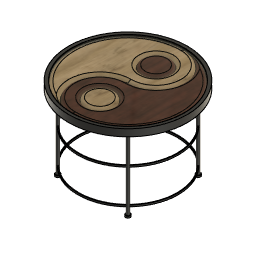
Yin+and+Yang+Table (Autodesk Fusion 360 design; units mm, degrees)
Autodesk Fusion 360 part; units mm, degrees
sketch "Sketch1" plane through (0, 0, 0) normal (0, 0, 1) x (1, 0, 0)
  circle A0 centre (0, 0) radius 457.2
  circle A1 centre (0, -228.6) radius 114.3
  circle A2 centre (0, 228.6) radius 114.3
  arc A3 (0, 0) -> (0, 457.2) centre (0, 228.6) ccw
  arc A4 (0, 0) -> (0, -457.2) centre (0, -228.6) ccw
  dimension "d5" = 457.2
  dimension "d6" = 457.2
  dimension "d7" = 228.6
  dimension "d8" = 228.6
  dimension "d9" = 228.6
  dimension "d10" = 228.6
  dimension "d11" = 914.4
  dimension "d12" = 228.6
  dimension "d13" = 228.6
  constraint coincident A0.centre A3.start
  constraint concentric A1 A4
  constraint concentric A2 A3
  constraint coincident A0 A3.end
  constraint coincident A0.centre A4
  constraint coincident A0 A4.end
  constraint coincident A3 A0.centre
  measures "d5" diameter of A3
  measures "d6" diameter of A4
  measures "d7" diameter of A1
  measures "d8" diameter of A2
  measures "d9" distance of A0.centre A2.centre
  measures "d10" distance of A0.centre A1.centre
  measures "d11" diameter of A0
  measures "d12" radius of A4
  measures "d13" radius of A3
extrude "Extrude1" add sketch "Sketch1" along normal blind 50.8 contours A0 A3 A4 | A1 picked at (-228.0212, 95.0056) makes body 1 at (-228.0212, 95.0056, 0) makes body 2 at (-59.3187, -250.0625, 0) in component "Component"
extrude "Extrude1'" add sketch "Sketch1" along normal blind 50.8 separate body contours A0 A3 A4 | A2 picked at (232.3828, -82.2636) makes body 3 at (228.0212, -95.0056, 0) makes body 4 at (35.0802, 259.2365, 0) in component "Component'"
fillet "Fillet1" radius 25.4 2 faces at (228.0212, -95.0056, 50.8) (35.0802, 259.2365, 50.8) on bodies 3 4 in component "Component'"
fillet "Fillet1'" radius 25.4 2 faces at (-228.0212, 95.0056, 50.8) (-59.3187, -250.0625, 50.8) on bodies 1 2 in component "Component"
sketch "Sketch2" plane through (0, 0, 0) normal (0, 0, 1) x (1, 0, 0)
  circle A0 centre (0, 0) radius 457.2
  circle A1 centre (0, 0) radius 482.6
  circle A2 centre (0, 0) radius 469.9
  dimension "d29" = 914.4
  dimension "d30" = 25.4
  dimension "d31" = 12.7
  constraint coincident A0.centre A1.centre
  measures "d29" diameter of A0
extrude "Extrude3" add sketch "Sketch2" along normal blind 57.15 separate body contours A1 | A2 makes body 5
extrude "Extrude4" add sketch "Sketch2" against normal blind 5.08 separate body contours A0 | A2 makes body 6
sketch "Sketch3" plane through (0, 0, 0) normal (0, 0, 1) x (1, 0, 0)
  circle A0 centre (0, 0) radius 457.2
  circle A1 centre (0, 0) radius 457.2
  line L0 (0, -457.2) -> (395.9468, -228.6)
  line L1 (395.9468, -228.6) -> (395.9468, 228.6)
  line L2 (395.9468, 228.6) -> (0, 457.2)
  line L3 (0, 457.2) -> (-395.9468, 228.6)
  line L4 (-395.9468, 228.6) -> (-395.9468, -228.6)
  line L5 (-395.9468, -228.6) -> (0, -457.2)
  line L6 (-370.5468, -213.9353) -> (0, -427.8706)
  line L7 (0, -427.8706) -> (370.5468, -213.9353)
  line L8 (370.5468, -213.9353) -> (370.5468, 213.9353)
  line L9 (370.5468, 213.9353) -> (0, 427.8706)
  line L10 (0, 427.8706) -> (-370.5468, 213.9353)
  line L11 (-370.5468, 213.9353) -> (-370.5468, -213.9353)
  line L12 (-345.1468, 199.2706) -> (-345.1468, -199.2706)
  line L13 (-345.1468, -199.2706) -> (0, -398.5412)
  line L14 (0, -398.5412) -> (345.1468, -199.2706)
  line L15 (345.1468, -199.2706) -> (345.1468, 199.2706)
  line L16 (345.1468, 199.2706) -> (0, 398.5412)
  line L17 (0, 398.5412) -> (-345.1468, 199.2706)
  line L18 (0, -50.8) -> (43.9941, -25.4)
  line L19 (43.9941, -25.4) -> (43.9941, 25.4)
  line L20 (43.9941, 25.4) -> (0, 50.8)
  line L21 (0, 50.8) -> (-43.9941, 25.4)
  line L22 (-43.9941, 25.4) -> (-43.9941, -25.4)
  line L23 (-43.9941, -25.4) -> (0, -50.8)
  dimension "d36" = 914.4
  dimension "d37" = 914.4
  dimension "d38" = -25.4
  dimension "d39" = -50.8
  dimension "d46" = 50.8
  constraint coincident A0.centre A1.centre
  constraint coincident A0 L0.start
  measures "d36" diameter of A0
  measures "d37" diameter of A1
  measures "d46" distance of L18.start A0.centre
extrude "Extrude5" add sketch "Sketch3" against normal blind 25.4 separate body contours L6 L7 L8 L9 L10 L11 makes body 7
sketch "Sketch4" plane through (0, 0, 0) normal (0, 0, 1) x (1, 0, 0)
  circle A0 centre (0, 0) radius 457.2
  line L0 (323.2892, 323.2892) -> (-323.2892, 323.2892)
  line L1 (-323.2892, 323.2892) -> (-323.2892, -323.2892)
  line L2 (-323.2892, -323.2892) -> (323.2892, -323.2892)
  line L3 (323.2892, -323.2892) -> (323.2892, 323.2892)
  line L4 (323.2892, 323.2892) -> (-323.2892, -323.2892) construction
  line L5 (-323.2892, 323.2892) -> (323.2892, -323.2892) construction
  dimension "d42" = 914.4
  dimension "d43" = 90
  constraint coincident A0.centre origin
  constraint horizontal L0
  constraint perpendicular L0 L1
  constraint parallel L0 L2
  constraint parallel L1 L3
  constraint coincident L4 A0.centre
  constraint coincident L5 A0.centre
  constraint coincident A0 L0.start
  measures "d42" diameter of A0
  measures "d43" angle of L4 L5
sketch "Sketch5" plane through (0, 0, 0) normal (0, 0, 1) x (1, 0, 0)
  circle A0 centre (0, 0) radius 457.2
  line L0 (0, 0) -> (-482.6, 0) construction
  dimension "d44" = 914.4
  constraint coincident A0.centre L0.start
  constraint horizontal L0
  measures "d44" diameter of A0
extrude "Extrude6" add sketch "Sketch3" against normal blind 609.6 separate body contours L18 L19 L20 L21 L22 L23 makes body 8
sketch "Sketch6" plane through (0, 0, 0) normal (0, 0, 1) x (1, 0, 0)
  line L0 (285.75, -285.75, -5.08) -> (-285.75, -285.75, -5.08)
  line L1 (-285.75, -285.75, -5.08) -> (-285.75, 285.75, -5.08)
  line L2 (-285.75, 285.75, -5.08) -> (285.75, 285.75, -5.08)
  line L3 (285.75, 285.75, -5.08) -> (285.75, -285.75, -5.08)
  line L4 (285.75, -285.75, -5.08) -> (-285.75, 285.75, -5.08) construction
  line L5 (-285.75, -285.75, -5.08) -> (285.75, 285.75, -5.08) construction
  line L6 (-285.75, 285.75, -5.08) -> (-260.35, 285.75, -5.08)
  line L7 (-260.35, 285.75, -5.08) -> (-260.35, 260.35, -5.08)
  line L8 (-260.35, 260.35, -5.08) -> (-285.75, 260.35, -5.08)
  line L9 (-285.75, 260.35, -5.08) -> (-285.75, 285.75, -5.08)
  line L10 (285.75, 285.75, -5.08) -> (260.35, 285.75, -5.08)
  line L11 (260.35, 285.75, -5.08) -> (260.35, 260.35, -5.08)
  line L12 (260.35, 260.35, -5.08) -> (285.75, 260.35, -5.08)
  line L13 (285.75, 260.35, -5.08) -> (285.75, 285.75, -5.08)
  line L14 (-285.75, -285.75, -5.08) -> (-212.2467, -285.75, -5.08)
  line L15 (-212.2467, -285.75, -5.08) -> (-212.2467, -212.2467, -5.08)
  line L16 (-212.2467, -212.2467, -5.08) -> (-285.75, -212.2467, -5.08)
  line L17 (-285.75, -212.2467, -5.08) -> (-285.75, -285.75, -5.08)
  line L18 (285.75, -285.75, -5.08) -> (210.9673, -285.75, -5.08)
  line L19 (210.9673, -285.75, -5.08) -> (210.9673, -210.9673, -5.08)
  line L20 (210.9673, -210.9673, -5.08) -> (285.75, -210.9673, -5.08)
  line L21 (285.75, -210.9673, -5.08) -> (285.75, -285.75, -5.08)
  circle A0 through (-273.05, -285.75, -5.08) (-292.1, -274.7515, -5.08) (-292.1, -296.7485, -5.08)
  circle A1 through (298.45, -285.75, -5.08) (279.4, -274.7515, -5.08) (279.4, -296.7485, -5.08)
  circle A2 through (-273.05, 285.75, -5.08) (-292.1, 296.7485, -5.08) (-292.1, 274.7515, -5.08)
  circle A3 through (298.45, 285.75, -5.08) (279.4, 296.7485, -5.08) (279.4, 274.7515, -5.08)
  circle A4 through (469.9, 0, -5.08) (-234.95, 406.9453, -5.08) (-234.95, -406.9453, -5.08)
  circle A5 centre (0, 0) radius 404.1115
  circle A6 centre (0, 0) radius 407.2865
  circle A7 centre (0, 0) radius 400.9365
  dimension "d49" = 571.5
  dimension "d50" = 571.5
  dimension "d51" = 25.4
  dimension "d52" = 25.4
  dimension "d53" = 25.4
  dimension "d54" = 25.4
  dimension "d55" = 25.4
  dimension "d59" = 25.4
  dimension "d60" = 25.4
  dimension "d62" = 25.4
  dimension "d68" = 3.175
  dimension "d69" = -3.175
  constraint coincident A5.centre A6.centre
extrude "Extrude1''" add sketch "Sketch6" against normal blind 609.6 separate body contours L0 L3 L18 L21 A1 | L0 L3 L18 L21 A1 | L0 L1 L14 L17 A0 | L0 L1 L14 L17 A0 | L2 L3 L10 L13 A3 | L2 L3 L10 L13 A3 | L1 L2 L6 L9 A2 | L1 L2 L6 L9 A2 in plane through (0, 0, -5.08) normal (0, 0, 1) makes body 9 at (298.0573, -288.8838, -208.28) makes body 10 at (-273.3018, -283.2335, -411.48) makes body 11 at (298.1982, 288.2665, -411.48) makes body 12 at (-273.3018, 288.2665, -411.48) in component "Component''"
copy_body "Body->Comp1" bodies 5 removing the originals makes body 13 in component "Component'''"
copy_body "CutPasteBodies1" bodies 6 removing the originals makes body 14 in component "Component'''"
sketch "Sketch7" plane through (0, 0, 57.15) normal (0, 0, 1) x (-1, 0, 0)
  circle A0 centre (0, 0) radius 457.2
  circle A1 centre (0, 0) radius 482.6
  circle A2 centre (0, 0) radius 457.2
extrude "Extrude7" add sketch "Sketch7" against normal blind 7.9375 from surface at -1.524 separate body contours A0 A2 makes body 15
sketch "Sketch8" plane through (0, 0, -614.68) normal (0, 0, -1) x (1, 0, 0)
  circle A0 centre (-285.75, -285.75) radius 12.7
  circle A1 centre (-285.75, -285.75) radius 19.05
  dimension "d65" = 38.1
  constraint concentric A0 A1
  measures "d65" diameter of A1
extrude "Extrude8" add sketch "Sketch8" against normal blind 12.7 separate body makes body 16
copy_body "CopyPasteBodies1" bodies 16 makes body 17
move_body "Move1" bodies 17 to x (1, 0, 0) y (0, 1, 0) z (0, 0, 1) at (0, -571.5, 0)
copy_body "CopyPasteBodies2" bodies 16 makes body 18
move_body "Move2" bodies 18 to x (1, 0, 0) y (0, 1, 0) z (0, 0, 1) at (571.5, -571.5, 0)
copy_body "CopyPasteBodies3" bodies 16 makes body 19
move_body "Move3" bodies 19 to x (1, 0, 0) y (0, 1, 0) z (0, 0, 1) at (571.5, 0, 0)
sketch "Sketch9" plane through (0, 0, 0) normal (0, 0, 1) x (1, 0, 0)
  circle A0 centre (0, 0) radius 407.2865
  circle A1 centre (0, 0) radius 404.1115
  circle A2 centre (0, 0) radius 400.9365
  dimension "d70" = 3.175
  dimension "d71" = -3.175
extrude "Extrude9" add sketch "Sketch9" against normal blind 12.7 from surface at -304.8 separate body contours A0 | A1 makes body 20
copy_body "CopyPasteBodies4" bodies 20 makes body 21
move_body "Move4" bodies 21 to x (1, 0, 0) y (0, 1, 0) z (0, 0, 1) at (0, 0, -254)
move_body "Move5" bodies 20 to x (1, 0, 0) y (0, 1, 0) z (0, 0, 1) at (0, 0, 50.8)
move_body "Move6" bodies 21 to x (1, 0, 0) y (0, 1, 0) z (0, 0, 1) at (0, 0, 25.4)
component "Component" placed x (1, 0, 0) y (0, 1, 0) z (0, 0, 1) at (0, 0, 0)
component "Component'" placed x (1, 0, 0) y (0, 1, 0) z (0, 0, 1) at (0, 0, 0)
component "Component''" placed x (1, 0, 0) y (0, 1, 0) z (0, 0, 1) at (0, 0, 0)
component "Component'''" placed x (1, 0, 0) y (0, 1, 0) z (0, 0, 1) at (0, 0, 0)
hidden bodies 7 8
equation "radius = 18 in"
equation "d5 = radius"
equation "d6 = radius"
equation "d7 = radius / 2"
equation "d8 = radius / 2"
equation "d9 = radius / 2"
equation "d10 = radius / 2"
equation "d11 = radius * 2"
equation "thic = 2 in"
equation "d17 = thic"
equation "d19 = thic"
equation "rond = 1 in"
equation "d23 = rond"
equation "d25 = rond"
equation "d29 = radius * 2"
equation "d36 = radius * 2"
equation "d37 = radius * 2"
equation "d42 = radius * 2"
equation "d44 = radius * 2"
equation "d49 = radius * 1.25"
equation "d50 = radius * 1.25"
equation "Tall = 24 in"
equation "d57 = -Tall"
equation "d63 = ( -5 / 16 ) * 1 in"
